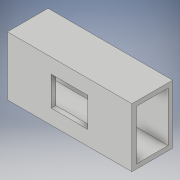
# Autodesk Inventor part: Scanner Case v3
Saved by Autodesk Inventor 2018 (Build 220112000, 112)
## iProperties
Created: 2018-04-04
Part Number: Scanner Case v3
Material: Generic
Document SubType Name: Modeling
Designer: arche
Density: 1 g/cm^3
Appearance: Default
Author: arche
Autodesk Inventor part; units mm, degrees
ref_plane "YZ Plane" through (0, 0, 0) normal (1, 0, 0) x (0, 1, 0)
ref_plane "XZ Plane" through (0, 0, 0) normal (0, 1, 0) x (-1, 0, 0)
ref_plane "XY Plane" through (0, 0, 0) normal (0, 0, 1) x (1, 0, 0)
sketch "Sketch1" plane through (0, 0, 0) normal (0, 0, 1) x (1, 0, 0)
  line L0 (0, 0) -> (-69.85, 0)
  line L1 (-69.85, 0) -> (-69.85, 33.02)
  line L2 (-69.85, 33.02) -> (0, 33.02)
  line L3 (0, 33.02) -> (0, 0)
  dimension "d0" = 69.85
  dimension "d1" = 33.02
  constraints: 8 end point, 2 parallel, 1 horizontal, 1 perpendicular
  measures "d0" distance of L1.end L2.end
  measures "d1" distance of L0.end L1.end
extrude "Extrusion1" add sketch "Sketch1" along normal blind 22.86
shell "Shell1" thickness 2.54 removed faces 1 at (0, 22.0133, 15.24)
sketch "Sketch2" plane through (0, 0, 22.86) normal (0, 0, 1) x (1, 0, 0)
  line L0 (0, 33.02) -> (-69.85, 33.02) projected
  line L1 (-69.85, 0) -> (0, 0) projected
  line L2 (-69.85, 33.02) -> (-69.85, 0) projected
  line L3 (0, 0) -> (0, 33.02) projected
  line L4 (-45.212, 16.51) -> (-45.212, 24.765)
  line L5 (-45.212, 24.765) -> (-34.925, 24.765)
  line L6 (-34.925, 8.255) -> (-45.212, 8.255)
  line L7 (-45.212, 8.255) -> (-45.212, 16.51)
  line L8 (-24.638, 16.51) -> (-24.638, 8.255)
  line L9 (-24.638, 8.255) -> (-34.925, 8.255)
  line L10 (-24.638, 16.51) -> (-24.638, 24.765)
  line L11 (-24.638, 24.765) -> (-34.925, 24.765)
  constraints: 16 end point, 3 point on line
extrude "Extrusion2" cut sketch "Sketch2" against normal blind 2.54 contours L4 L5 L11 L10 L8 L9 L6 L7
body "Solid1"
